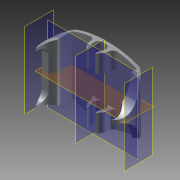
# Autodesk Inventor part: chasis
Saved by Autodesk Inventor 2012 (Build 160160000, 160)
## iProperties
Created: 2012-12-28
Part Number: chasis
Material: Default
Document SubType Name: Modeling
Designer: otrebor
Density: 1 g/cm^3
Author: otrebor
Autodesk Inventor part; units mm, degrees
ref_plane "YZ Plane" through (0, 0, 0) normal (1, 0, 0) x (0, 1, 0)
ref_plane "XZ Plane" through (0, 0, 0) normal (0, 1, 0) x (-1, 0, 0)
ref_plane "XY Plane" through (0, 0, 0) normal (0, 0, 1) x (1, 0, 0)
sketch "Boceto1" plane through (0, 0, 0) normal (0, 0, 1) x (1, 0, 0)
  line L0 (-3.4214, 5.0502) -> (3.4219, 5.0498)
  line L1 (-3.4219, -5.0498) -> (3.4214, -5.0502)
  arc A0 (-3.4214, 5.0502) -> (-3.4219, -5.0498) centre (0, 0) ccw
  arc A1 (3.4214, -5.0502) -> (3.4219, 5.0498) centre (0, 0) ccw
  line L2 (-4.2144, -8.0498) -> (4.2598, -8.0502)
  arc A2 (-9.0862, 0.0316) -> (-4.2144, -8.0498) centre (0, 0) ccw
  arc A3 (4.2598, -8.0502) -> (9.1077, 0.0307) centre (0, 0) ccw
  line L3 (-18.1683, 5.0493) -> (-14.0859, 5.049)
  line L4 (-18.1683, 5.0493) -> (-32.9096, 5.05)
  arc A4 (14.108, 5.0476) -> (9.1077, 0.0307) centre (14.1077, 0.0476) ccw
  arc A5 (-9.0862, 0.0316) -> (-14.0859, 5.049) centre (-14.0862, 0.049) ccw
  line L5 (55.8573, -11.007) -> (-54.3124, -11.0015) construction
  line L6 (0.0842, 24.332) -> (0.0818, -24.0148) construction
  line L7 (0.0821, -18.05) -> (-38.3243, -25.6599) construction
  line L8 (-21.9182, -22.4092) -> (-21.9159, 22.2845) construction
  line L9 (-21.9159, 22.2845) -> (-21.9164, 12.8414) construction
  arc A6 (-32.9166, 8.05) -> (-38.3243, -25.6599) centre (-21.9176, -11.0031) ccw
  arc A7 (-32.9104, -9.8037) -> (-38.3243, -25.6599) centre (-21.9182, -22.4092) ccw
  line L10 (-32.9096, 5.05) -> (-32.9104, -9.8037)
  arc A8 (38.4876, -25.6638) -> (33.0834, 8.0467) centre (22.0824, -11.0053) ccw
  arc A9 (38.4876, -25.6638) -> (33.0753, -9.807) centre (22.0818, -22.4114) ccw
  line L11 (33.0761, 5.0467) -> (33.0753, -9.807)
  line L12 (14.108, 5.0476) -> (33.0761, 5.0467)
  line L13 (33.0834, 8.0467) -> (-32.9166, 8.05)
  point P0 (-7.5545, 5.0487)
  point P1 (7.5766, 5.0543)
  dimension "d2" = 5.05
  dimension "d4" = 5.05
  dimension "d9" = 3
  dimension "d13" = 5
  dimension "d14" = 5
  dimension "d19" = 22
  dimension "d20" = 10
  dimension "d21" = 66
  dimension "d22" = 22
  dimension "d23" = 16.725
  dimension "d24" = 3
  constraints: 28 end point, 23 point on circle, 10 centre point, 6 point on line, 6 symmetric about line, 4 parallel, 4 tangent, 3 coincident, 2 perpendicular, 1 collinear, 3 other
  measures "d2" distance from line of L0 point (0, 0)
  measures "d4" distance from line of L1 point (0, 0)
  measures "d9" distance between parallel lines of L2 L1
  measures "d13" radius of A4
  measures "d14" radius of A5
  measures "d19" distance between parallel lines of L6 L8
  measures "d20" distance from line of L7.start L2
  measures "d21" distance of L13.start L13.end
  measures "d22" radius of A6
  measures "d23" radius of A7
  measures "d24" distance between parallel lines of L4 L13
extrude "Extrusión1" add sketch "Boceto1" along normal blind 70
ref_plane "Plano de trabajo1" through (0, 0, 35) normal (0, 0, 1) x (1, 0, 0)
sketch "Boceto2" plane through (0, 0, 35) normal (0, 0, 1) x (1, 0, 0)
  line L0 (-14.0895, -8.6113) -> (14.0431, -8.6113)
  line L1 (14.0431, -8.6113) -> (14.0431, 5.0579)
  line L2 (14.0431, 5.0579) -> (-14.0895, 5.0579)
  line L3 (-14.0895, 5.0579) -> (-14.0895, -8.6113)
  point P0 (0, 0)
  constraints: 8 end point, 2 parallel, 1 horizontal, 1 perpendicular
extrude "Extrusión2" cut sketch "Boceto2" along normal mid plane 34
ref_plane "Plano de trabajo2" through (0.0825, -9.8053, 0) normal (-1, 0.0000505, 0) x (0, 0, 1)
ref_plane "Plano de trabajo3" through (49.0825, -9.8078, 0) normal (-1, 0.0000505, 0) x (0, 0, 1)
sketch "Boceto3" plane through (49.0825, -9.8078, 0) normal (-1, 0.0000505, 0) x (0, 0, 1)
  ellipse E0 centre (0, -12.627) end of major axis (33, -12.627) minor radius 23
  line L0 (35.0136, 0.2712) -> (35.0136, 5.1423) construction
  ellipse E1 centre (70.0272, -12.627) end of major axis (37.0272, -12.627) minor radius 23
  point P0 (0, 9.8053)
  dimension "d33" = 23
  dimension "d34" = 33
  constraints: 2 end point, 2 vertical, 1 symmetric about line, 4 other
extrude "Extrusión3" cut sketch "Boceto3" along normal blind 34
ref_plane "Plano de trabajo4" through (-3.422, -6.5498, 0) normal (0.0000505, 1, 0) x (1, -0.0000505, 0)
sketch "Boceto4" plane through (-4.2144, -8.0498, 70) normal (-0.0000505, -1, 0) x (1, -0.0000505, 0)
  line L0 (0, 0) -> (8.4742, 0)
  line L1 (8.4742, 0) -> (8.4742, -18)
  line L2 (8.4742, -18) -> (0, -18)
  line L3 (0, -18) -> (0, 0)
  line L4 (0, -18) -> (0, 0) projected
  line L5 (-6.0414, -34.9865) -> (12.2384, -34.9865)
  point P0 (4.214, -70)
  constraints: 10 end point, 2 parallel, 2 perpendicular, 1 horizontal
extrude "Extrusión4" cut sketch "Boceto4" against normal blind 4
sketch "Boceto5" plane through (-4.2144, -8.0498, 0) normal (-0.0000505, -1, 0) x (1, -0.0000505, 0)
  line L0 (0, 18) -> (8.4742, 18)
  line L1 (8.4742, 18) -> (8.4742, 0)
  line L2 (8.4742, 0) -> (0, 0)
  line L3 (0, 0) -> (0, 18)
  point P0 (4.214, 0)
  constraints: 8 end point, 2 parallel, 1 horizontal, 1 perpendicular
extrude "Extrusión5" cut sketch "Boceto5" against normal blind 4
sketch "Boceto6" plane through (-32.9166, 8.05, 0) normal (0.0000505, 1, 0) x (1, -0.0000505, 0)
  line L0 (0, 0) -> (0, -70) projected
  line L1 (32.9166, 8.272) -> (32.9166, -95.5522) construction
  line L2 (-17.5554, -35) -> (113.403, -35) construction
  ellipse E0 centre (32.9166, -35) end of major axis (91.2554, -35) minor radius 35.21
  point P0 (32.917, 0)
  constraints: 4 end point, 2 point on line, 1 parallel, 1 perpendicular, 2 other
extrude "Extrusión6" cut sketch "Boceto6" against normal blind 35.75 keep common part
ref_plane "Plano de trabajo5" through (-51.4175, -9.8027, 0) normal (-1, 0.0000505, 0) x (0, 0, 1)
sketch "Boceto7" plane through (-51.4175, -9.8027, 0) normal (-1, 0.0000505, 0) x (0, 0, 1)
  arc A0 (18.5655, -4.9415) -> (11.2138, -12.2932) centre (18.5655, -12.2932) ccw
  line L0 (34.9889, 15.9835) -> (34.9889, -24.1466) construction
  line L1 (18.5655, -4.9415) -> (34.9889, -4.9415)
  arc A1 (58.7638, -12.3305) -> (51.4122, -4.9415) centre (51.4122, -12.2932) ccw
  line L2 (51.4122, -4.9415) -> (34.9889, -4.9415)
  line L3 (11.2138, -12.2932) -> (11.2138, -16.4437)
  line L4 (11.2138, -16.4437) -> (58.7638, -16.4437)
  line L5 (58.7638, -12.3305) -> (58.7638, -16.4437)
  point P0 (0, 9.8053)
  point P1 (34.9889, -15.3035)
  point P2 (11.8584, -15.3035)
  point P3 (58.1193, -15.3035)
  constraints: 12 end point, 4 point on circle, 3 perpendicular, 3 symmetric about line, 2 centre point, 2 point on line, 2 tangent, 1 vertical, 1 other
extrude "Extrusión7" cut sketch "Boceto7" against normal blind 24.75
equation "\"d4\" = d2"
equation "\"d9\" = d8"
equation "\"d19\" = 0.333333 * d21"
equation "\"d8\" = 3"
